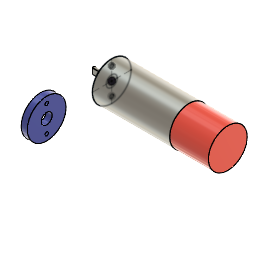
MOTOR (Autodesk Fusion 360 design; units mm, degrees)
part number: 2025-10-04-12-29-30-471
part number: 2025-10-04-14-22-54-438
part number: 2025-10-04-14-23-30-722
Autodesk Fusion 360 part; units mm, degrees
sketch "Sketch1" plane through (0, 0, 0) normal (1, 0, 0) x (0, 1, 0)
  circle A0 centre (0, 0) radius 12.5
  circle A1 centre (0, 8.5) radius 1.1
  line L0 (0, 0) -> (0, -12.5) construction
  line L1 (0, 0) -> (0, 12.5) construction
  line L2 (0, 0) -> (-12.5, 0) construction
  line L3 (0, 0) -> (12.5, 0) construction
  circle A2 centre (0, -8.5) radius 1.1
  circle A3 centre (0, 0) radius 3.5
  circle A4 centre (0, 0) radius 2
  dimension "d1" = 25
  dimension "d2" = 2.2
  dimension "d3" = 8.5
  dimension "d4" = 7
  dimension "d5" = 4
  constraint coincident A0.centre L0.start
  constraint coincident A0 L0.end
  constraint vertical L0
  constraint coincident A0 L1.end
  constraint parallel L0 L1
  constraint coincident A1.centre L1
  constraint coincident A0 L2.end
  constraint perpendicular L0 L2
  constraint coincident A0 L3.end
  constraint perpendicular L0 L3
  constraint symmetric A1 L3 A2
  constraint concentric A0 A3
  measures "d1" diameter of A0
  measures "d2" diameter of A1
  measures "d3" vertical distance of A0.centre A1.centre
  measures "d4" diameter of A3
  measures "d5" diameter of A4
extrude "Extrude1" add sketch "Sketch1" along normal blind 50 contours A0 | A1 | A2 | A3 | A4 makes body 1
extrude "Extrude2" add sketch "Sketch1" against normal blind 2.5 contours A3 bodies 1
extrude "Extrude3" add sketch "Sketch1" against normal blind 12 contours A4 bodies 1
extrude "Extrude4" cut sketch "Sketch1" along normal blind 9 contours A1 | A2 bodies 1
box "BoxPrimitive1" cut length 3.751 width 2 height -8 placed x (0, 0, -1) y (0, -1, 0) z (-1, 0, 0) at (-12, -0.6146, 1.8474) bodies 1
extrude "Extrude1'" add sketch "Sketch1" against normal blind 4 separate body contours A0 makes body 2 in component "CAP1"
move_body "Move1" bodies 2 to x (1, 0, 0) y (0, 1, 0) z (0, 0, 1) at (0, -42, 0) in component "CAP1"
copy_body "Body->Comp1" bodies 1 removing the originals makes body 3 in component "MOTOR"
hole "Hole1" at (-4, -42, 8.5) direction (1, 0, 0) diameter 1.8 depth 12 tip angle 118 countersink diameter 3.5 countersink angle 90 bodies 2 in component "CAP1"
hole "Hole2" at (-4, -42, -8.5) direction (1, 0, 0) diameter 2.2 depth 119.79 tip angle 118 countersink diameter 3.5 countersink angle 90 bodies 2 in component "CAP1"
cylinder "CylinderPrimitive1" add diameter 25 height 25 placed x (0, 0, -1) y (0, 1, 0) z (1, 0, 0) at (50, 0, 0) separate body makes body 4 in component "MOTOR"
component "CAP1" placed x (1, 0, 0) y (0, 1, 0) z (0, 0, 1) at (0, 0, 0)
component "MOTOR" placed x (1, 0, 0) y (0, 1, 0) z (0, 0, 1) at (0, 0, 0)
named bodies: "CAP", "MOTOR"
